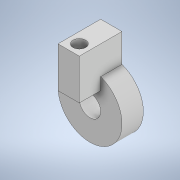
# Autodesk Inventor part: End motor link
Saved by Autodesk Inventor 2022 (Build 260153000, 153)
## iProperties
Created: 2022-01-28
Part Number: End motor link
Material: Generic
Document SubType Name: Modeling
Designer: Alexa
Density: 1 g/cm^3
Appearance: Default
Author: Alexa
Autodesk Inventor part; units mm, degrees
ref_plane "YZ Plane" through (0, 0, 0) normal (1, 0, 0) x (0, 1, 0)
ref_plane "XZ Plane" through (0, 0, 0) normal (0, 1, 0) x (-1, 0, 0)
ref_plane "XY Plane" through (0, 0, 0) normal (0, 0, 1) x (1, 0, 0)
sketch "Sketch1" plane through (0, 0, 0) normal (0, 0, 1) x (1, 0, 0)
  circle A0 centre (0, 0) radius 30
  circle A1 centre (0, 0) radius 10
  line L0 (-30, 0) -> (30, 0)
  line L1 (30, 0) -> (30, 20)
  line L2 (30, 20) -> (-30, 20)
  line L3 (-30, 20) -> (-30, 0)
  line L4 (-10, 20) -> (10, 20)
  line L5 (10, 20) -> (10, 55)
  line L6 (10, 55) -> (-10, 55)
  line L7 (-10, 55) -> (-10, 20)
  point P0 (10, 28.2843)
  point P1 (-10, 28.2843)
  dimension "d0" = 60
  dimension "d1" = 20
  dimension "d2" = 20
  dimension "d3" = 20
  dimension "d4" = 35
  constraints: 16 end point, 4 parallel, 2 coincident, 2 horizontal, 2 perpendicular, 1 centre point, 1 point on line, 3 other
  measures "d1" diameter of A1
  measures "d2" distance of L1.end L0.end
  measures "d3" distance of L6.end L5.end
  measures "d4" distance of L5.end L4.end
extrude "Extrusion1" add sketch "Sketch1" along normal blind 40 contours L0 A1 A0 | A0 L2 L0 A1 | A0 L7 L2 | L2 L5 A0 | L7 L6 L5 A0 | A0 L5 L2 L7
sketch "Sketch2" plane through (0, 0, 40) normal (0, 0, 1) x (1, 0, 0)
  circle A0 centre (0, 0) radius 30
  line L0 (10, 55) -> (-10, 55) projected
  line L1 (-10, 55) -> (10, 55)
  line L2 (10, 55) -> (10, 17)
  line L3 (10, 17) -> (-10, 17)
  line L4 (-10, 17) -> (-10, 55)
  circle A1 centre (0, 0) radius 10
  point P0 (-10, 28.2843)
  point P1 (10, 28.2843)
  dimension "d7" = 38
  constraints: 8 end point, 2 centre point, 2 coincident, 2 parallel, 1 horizontal, 1 perpendicular
  measures "d7" distance of L1.end L2.end
extrude "Extrusion2" cut sketch "Sketch2" against normal blind 20 contours A0 L4 L3 L2 picked at (15.0969, 11.943)
sketch "Sketch3" plane through (-10, 55, 0) normal (0, 1, 0) x (1, 0, 0)
  circle A0 centre (10, -30) radius 6
  point P0 (10, 0)
  dimension "d10" = 12
  constraints: 1 centre point
  measures "d10" diameter of A0
extrude "Extrusion3" cut sketch "Sketch3" against normal blind 40.325
body "Solid1"
